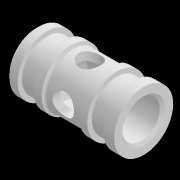
# Autodesk Inventor part: checkBallValve
Saved by Autodesk Inventor 2021 (Build 250183000, 183)
## iProperties
Created: 2024-03-20
Part Number: checkBallValve
Material: Generic
Document SubType Name: Modeling
Designer: top10
Density: 1 g/cm^3
Appearance: Default
Author: top10
Autodesk Inventor part; units mm, degrees
ref_plane "YZ Plane" through (0, 0, 0) normal (1, 0, 0) x (0, 1, 0)
ref_plane "XZ Plane" through (0, 0, 0) normal (0, 1, 0) x (-1, 0, 0)
ref_plane "XY Plane" through (0, 0, 0) normal (0, 0, 1) x (1, 0, 0)
sketch "Sketch2" plane through (0, 0, 0) normal (0, 0, 1) x (1, 0, 0)
  line L0 (0, 9.2393) -> (0, -9.2393) construction
  line L1 (-14.831, 0) -> (14.831, 0)
  line L2 (-10, 5.5) -> (10, 5.5)
  line L3 (10, 5.5) -> (10, 3.5)
  line L4 (10, 3.5) -> (-4, 3.5)
  line L5 (-4, 3.5) -> (-6, 2.5)
  line L6 (-6, 2.5) -> (-10, 2.5)
  line L7 (-10, 2.5) -> (-10, 5.5)
  circle A0 centre (-2.75, 0) radius 3.75 construction
  line L8 (-8, 5.5) -> (-5, 5.5)
  line L9 (-5, 5.5) -> (-5, 4.65)
  line L10 (-5, 4.65) -> (-8, 4.65)
  line L11 (-8, 4.65) -> (-8, 5.5)
  line L12 (5, 4.65) -> (8, 4.65)
  line L13 (8, 4.65) -> (8, 5.5)
  line L14 (8, 5.5) -> (5, 5.5)
  line L15 (5, 5.5) -> (5, 4.65)
  line L16 (-3.5, 5.5) -> (3.5, 5.5)
  line L17 (3.5, 5.5) -> (3.5, 5)
  line L18 (3.5, 5) -> (-3.5, 5)
  line L19 (-3.5, 5) -> (-3.5, 5.5)
  point P0 (0, 0)
  point P1 (0, 0)
  point P2 (-5, 3)
  point P3 (-5, 5.5)
  point P4 (3.5, 5.5)
  point P5 (0, 5.5)
  dimension "d6" = 7.5
  dimension "d0" = 7
  dimension "d1" = 11
  dimension "d2" = 10
  dimension "d3" = 10
  dimension "d5" = 5
  dimension "d7" = 6
  dimension "d8" = 4
  dimension "d11" = 2
  dimension "d12" = 3
  dimension "d13" = 9.3
  dimension "d14" = 9.3
  dimension "d15" = 3
  dimension "d16" = 2
  dimension "d31" = 7
  dimension "d32" = 0.5
  dimension "d34" = 1.15
  dimension "d35" = 1.5
  constraints: 40 end point, 7 horizontal, 6 point on line, 5 parallel, 5 perpendicular, 4 midpoint, 4 vertical, 2 coincident, 8 other
  measures "d0" diameter of L4 L1
  measures "d1" diameter of L2 L1
  measures "d2" distance between parallel lines of L0 L3
  measures "d3" distance between parallel lines of L0 L7
  measures "d5" diameter of L6 L1
  measures "d7" horizontal distance of L6.end L4.end
  measures "d8" distance of L6.end L5.end
  measures "d11" distance between parallel lines of L7 L11
  measures "d12" distance between parallel lines of L9 L11
  measures "d13" diameter of L10 L1
  measures "d14" diameter of L12 L1
  measures "d15" distance between parallel lines of L13 L15
  measures "d16" distance of L2.end L13.end
  measures "d31" distance of L17.end L18.end
  measures "d32" distance between parallel lines of L16 L18
  measures "d34" distance between parallel lines of L12 L4
  measures "d35" distance between parallel lines of L15 L17
revolve "Revolution1" add sketch "Sketch2" angle 360 about axis through (-14.831, 0, 0) along (1, 0, 0) contours L2 L11 L10 L9 L19 L18 L17 L15 L12 L13 L3 L4 L5 L6 L7
chamfer "Chamfer1" distance 0.5 angle 45 3 edges at (-10, -5.5, 0) (-10, -2.5, 0) (10, -3.5, 0)
ref_plane "Work Plane1" through (0, 5.5, 0) normal (0, 1, 0) x (-1, 0, 0)
sketch "Sketch3" plane through (0, 5.5, 0) normal (0, 1, 0) x (-1, 0, 0)
  point P0 (0, 0)
  point P1 (11, -4.7443)
hole "Hole1" at (0, 5.5, 0) direction (0, -1, 0) diameter 4 depth 15 tip angle 118
pattern_circular "Circular Pattern1" count 4 over 360 about axis through (3, 0, 0) along (1, 0, 0) of "Hole1"
fillet "Fillet1" radius 0.5 2 edges at (-3.5, -5, 0) (3.5, -5, 0)
equation "\"d14\" = d13"
equation "\"d15\" = d12"
body "Solid1"
